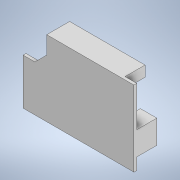
# Autodesk Inventor part: PD board supporter
Saved by Autodesk Inventor 2021 (Build 250183000, 183)
## iProperties
Created: 2022-01-29
Part Number: PD board supporter
Material: Generic
Document SubType Name: Modeling
Designer: Toby
Density: 1 g/cm^3
Appearance: Default
Author: Toby
Autodesk Inventor part; units mm, degrees
ref_plane "YZ Plane" through (0, 0, 0) normal (1, 0, 0) x (0, 1, 0)
ref_plane "XZ Plane" through (0, 0, 0) normal (0, 1, 0) x (-1, 0, 0)
ref_plane "XY Plane" through (0, 0, 0) normal (0, 0, 1) x (1, 0, 0)
sketch "Sketch1" plane through (0, 0, 0) normal (0, 0, 1) x (1, 0, 0)
  line L0 (-30.479, 15.7185) -> (11.521, 15.7185)
  line L1 (11.521, 15.7185) -> (11.521, 11.2185)
  line L2 (11.521, 11.2185) -> (-30.479, 11.2185)
  line L3 (-30.479, 11.2185) -> (-30.479, 15.7185)
  line L4 (-30.479, 11.2185) -> (-1.479, 11.2185)
  line L5 (-1.479, 11.2185) -> (-1.479, 3.2185)
  line L6 (-1.479, 3.2185) -> (-30.479, 3.2185)
  line L7 (-30.479, 3.2185) -> (-30.479, 11.2185)
  point P0 (0, 0)
  point P1 (-1.479, 11.2185)
  dimension "d0" = 42
  dimension "d1" = 4.5
  dimension "d2" = 29
  dimension "d3" = 8
  constraints: 16 end point, 4 parallel, 2 horizontal, 2 perpendicular
  measures "d0" distance of L0.start L0.end
  measures "d1" distance of L2.end L0.start
  measures "d2" distance of L5.end L6.end
  measures "d3" distance between parallel lines of L6 L2
extrude "Extrusion1" add sketch "Sketch1" along normal blind 8.5
sketch "Sketch2" plane through (0, 0, 8.5) normal (0, 0, 1) x (1, 0, 0)
  line L0 (-30.479, 15.7185) -> (-30.479, 3.2185) projected
  line L1 (-30.479, 15.7185) -> (16.521, 15.7185)
  line L2 (16.521, 15.7185) -> (16.521, -16.2815)
  line L3 (16.521, -16.2815) -> (-30.479, -16.2815)
  line L4 (-30.479, -16.2815) -> (-30.479, 15.7185)
  point P0 (0, 0)
  dimension "d6" = 47
  dimension "d7" = 32
  constraints: 8 end point, 2 parallel, 1 horizontal, 1 perpendicular
  measures "d6" distance of L2.end L3.end
  measures "d7" distance of L3.end L0.start
extrude "Extrusion2" add sketch "Sketch2" along normal blind 1.2
sketch "Sketch3" plane through (0, 0, 8.5) normal (0, 0, -1) x (-1, 0, 0)
  line L0 (30.479, 3.2185) -> (30.479, -16.2815) projected
  line L1 (30.479, -6.2815) -> (15.479, -6.2815)
  line L2 (15.479, -6.2815) -> (15.479, -13.2815)
  line L3 (15.479, -13.2815) -> (30.479, -13.2815)
  line L4 (30.479, -13.2815) -> (30.479, -6.2815)
  line L5 (30.479, -16.2815) -> (-16.521, -16.2815) projected
  point P0 (0, 0)
  dimension "d10" = 3
  dimension "d11" = 7
  dimension "d12" = 15
  constraints: 8 end point, 2 parallel, 1 horizontal, 1 perpendicular, 1 point on line
  measures "d10" distance between parallel lines of L5 L3
  measures "d11" distance between parallel lines of L3 L1
  measures "d12" distance of L1.start L1.end
extrude "Extrusion3" add sketch "Sketch3" along normal blind 8.5
sketch "Sketch4" plane through (0, 0, 8.5) normal (0, 0, -1) x (-1, 0, 0)
  line L0 (-16.521, -16.2815) -> (-16.521, 15.7185) projected
  line L1 (-16.521, -1.2815) -> (-9.521, -1.2815)
  line L2 (-9.521, -1.2815) -> (-9.521, -11.2815)
  line L3 (-9.521, -11.2815) -> (-16.521, -11.2815)
  line L4 (-16.521, -11.2815) -> (-16.521, -1.2815)
  line L5 (30.479, -16.2815) -> (-16.521, -16.2815) projected
  point P0 (0, 0)
  dimension "d15" = 7
  dimension "d16" = 10
  dimension "d17" = 5
  constraints: 8 end point, 2 parallel, 1 horizontal, 1 perpendicular, 1 point on line
  measures "d15" distance of L1.start L1.end
  measures "d16" distance of L1.end L2.end
  measures "d17" distance between parallel lines of L5 L3
extrude "Extrusion4" add sketch "Sketch4" along normal blind 8.5
sketch "Sketch5" plane through (0, 0, 0) normal (0, 0, -1) x (-1, 0, 0)
  line L0 (-16.521, 15.7185) -> (30.479, 15.7185) projected
  line L1 (30.479, 3.2185) -> (1.479, 3.2185) projected
  line L2 (30.479, 15.7185) -> (20.479, 15.7185)
  line L3 (20.479, 15.7185) -> (20.479, 3.2185)
  line L4 (20.479, 3.2185) -> (30.479, 3.2185)
  line L5 (30.479, 3.2185) -> (30.479, 15.7185)
  point P0 (0, 0)
  dimension "d20" = 10
  constraints: 8 end point, 2 parallel, 1 horizontal, 1 perpendicular, 1 point on line
  measures "d20" distance between parallel lines of L5 L3
extrude "Extrusion5" cut sketch "Sketch5" against normal blind 8.5
sketch "Sketch6" plane through (0, 0, 0) normal (0, 0, -1) x (-1, 0, 0)
  line L0 (15.479, -6.2815) -> (30.479, -6.2815) projected
  line L1 (15.479, -6.2815) -> (30.479, -6.2815)
  line L2 (30.479, -6.2815) -> (30.479, -9.2815)
  line L3 (30.479, -9.2815) -> (15.479, -9.2815)
  line L4 (15.479, -9.2815) -> (15.479, -6.2815)
  line L5 (30.479, -13.2815) -> (30.479, -6.2815) projected
  point P0 (0, 0)
  dimension "d23" = 3
  constraints: 8 end point, 2 parallel, 1 collinear, 1 horizontal, 1 perpendicular
  measures "d23" distance between parallel lines of L0 L3
extrude "Extrusion6" cut sketch "Sketch6" against normal blind 8.5
sketch "Sketch7" plane through (0, 0, 8.5) normal (0, 0, -1) x (-1, 0, 0)
  line L0 (-16.521, 15.7185) -> (30.479, 15.7185) projected
  line L1 (20.479, 15.7185) -> (30.479, 15.7185)
  line L2 (30.479, 15.7185) -> (30.479, 3.2185)
  line L3 (30.479, 3.2185) -> (20.479, 3.2185)
  line L4 (20.479, 3.2185) -> (20.479, 15.7185)
  line L5 (20.479, 3.2185) -> (1.479, 3.2185) projected
  line L6 (30.479, 15.7185) -> (30.479, -9.2815) projected
  line L7 (20.479, 3.2185) -> (20.479, 15.7185) projected
  point P0 (0, 0)
  constraints: 8 end point, 3 collinear, 2 parallel, 1 horizontal, 1 perpendicular, 1 point on line
extrude "Extrusion7" cut sketch "Sketch7" against normal blind 8.5
chamfer "Chamfer1" distance 5 angle 45 1 edges at (-20.479, 3.2185, 9.1)
body "Solid1"
